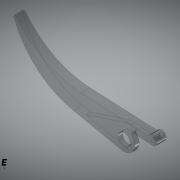
# Autodesk Inventor part: 後ろウイング先端
Saved by Autodesk Inventor 2020 (Build 240168000, 168)
## iProperties
Created: 2019-12-28
Part Number: 後ろウイング先端
Material: ポリカーボネート、クリア
Document SubType Name: Modeling
Designer: tanjihayato
Density: 1.2 g/cm^3
Appearance: ポリカーボネート - クリア
Author: tanjihayato
Autodesk Inventor part; units mm, degrees
ref_plane "YZ Plane" through (0, 0, 0) normal (1, 0, 0) x (0, 1, 0)
ref_plane "XZ Plane" through (0, 0, 0) normal (0, 1, 0) x (-1, 0, 0)
ref_plane "XY Plane" through (0, 0, 0) normal (0, 0, 1) x (1, 0, 0)
sketch "スケッチ1" plane through (0, 0, 0) normal (0, 0, 1) x (1, 0, 0)
  circle A0 centre (-145.5257, 0.5882) radius 1.5
  circle A1 centre (-139.5445, -10.0968) radius 1.5
  circle A2 centre (-105.5257, -16.4118) radius 30.1 construction
  line L0 (-170.915, -81.4118) -> (490.0044, -81.4118)
  circle A3 centre (-145.5257, 0.5882) radius 4.025
  circle A4 centre (-139.5445, -10.0968) radius 3
  circle A5 centre (-145.5257, 0.5882) radius 7.025
  line L1 (-146.2365, -6.4007) -> (-139.241, -7.1122)
  line L2 (-139.2044, 3.6529) -> (-134.6999, -5.6381)
  line L3 (-134.6999, -5.6381) -> (-136.7303, -11.1361)
  circle A6 centre (-105.5257, -16.4118) radius 31.1 construction
  line L4 (-145.1707, 7.6042) -> (-218.0775, 11.2924)
  line L5 (-145.8806, -6.4278) -> (-218.7874, -2.7396)
  circle A7 centre (-218.4324, 4.2764) radius 1.5
  circle A8 centre (-218.4324, 4.2764) radius 4.025
  circle A9 centre (-218.4324, 4.2764) radius 7.025
  circle A10 centre (-218.4324, 4.2764) radius 7.525
  line L6 (-214.5805, 10.7408) -> (-189.4684, -4.2228)
  circle A11 centre (-199.4194, 13.3524) radius 1.25
  arc A12 (-199.5709, 10.3562) -> (-202.1936, 14.494) centre (-199.4194, 13.3524) ccw
  line L7 (-202.1936, 14.494) -> (-247.2482, 16.7732)
  arc A13 (-289.8377, 39.1951) -> (-247.2482, 16.7732) centre (-244.3571, 73.9244) ccw
  arc A14 (-289.8377, 39.1951) -> (-291.571, 38.2429) centre (-290.6325, 38.5882) ccw
  arc A15 (-291.571, 38.2429) -> (-252.1456, 4.177) centre (-241.0929, 56.8157) ccw
  line L8 (-252.1456, 4.177) -> (-219.876, -2.5987)
  line L9 (-217.2943, 11.7148) -> (-212.7833, 11.0246)
  arc A16 (-212.7833, 11.0246) -> (-213.5315, 9.3094) centre (-212.8339, 10.0259) ccw
  line L10 (-220.7856, 11.424) -> (-246.4378, 2.9786)
  point P0 (0, 0)
  point P1 (0, 0)
  point P2 (0, 0)
  dimension "d17" = 6
  dimension "d18" = 8.05
  dimension "d19" = 3
  dimension "d20" = 1
  dimension "d21" = 3
  dimension "d22" = 8.05
  dimension "d23" = 3
  dimension "d24" = 0.5
  dimension "d25" = 2.5
  dimension "d26" = 6
  dimension "d27" = 2
  dimension "d28" = 120
  dimension "d29" = 4
  dimension "d30" = 150
  dimension "d31" = 1
  dimension "d32" = 73
  dimension "d33" = 79.9384
  constraints: 23 point on circle, 22 end point, 19 tangent, 16 centre point, 4 coincident, 4 point on line, 1 parallel, 4 other
  measures "d17" diameter of A4
  measures "d18" diameter of A3
  measures "d19" radial gap between concentric circles of A3 A5
  measures "d21" diameter of A7
  measures "d22" diameter of A8
  measures "d23" radial gap between concentric circles of A8 A9
  measures "d24" radial gap between concentric circles of A9 A10
  measures "d25" diameter of A11
  measures "d26" diameter of A12
  measures "d27" diameter of A14
  measures "d28" distance from line of L0 A14.centre
  measures "d29" distance between parallel lines of L4 L7
  measures "d30" distance of A14.centre A0.centre
  measures "d31" radius of A16
  measures "d32" distance of A0.centre A7.centre
  measures "d33" distance of A14.centre A7.centre
extrude "押し出し1" add sketch "スケッチ1" along normal blind 6 contours A16 A10 L6 | L6 A10 L4 A16 | L4 L9 A10 L10 L8 A15 A14 A13 L7 A12 | A9 | L8 L10 A10 | A10 L4 A9 L8 | A10 A16 A9 L4 | L4 A10 L9
extrude "押し出し2" cut sketch "スケッチ1" along normal blind 3 contours A16 A10 L6 | L6 A10 L4 A16 | A9 | L8 L10 A10 | A10 L4 A9 L8 | A10 A16 A9 L4 | L4 A10 L9
sketch "スケッチ2" plane through (0, 0, 0) normal (0, 0, -1) x (-1, 0, 0)
  circle A0 centre (199.4194, 13.3524) radius 1.25 projected
  line L0 (212.7833, 11.0246) -> (217.2943, 11.7148) projected
  arc A1 (220.7856, 11.424) -> (217.2943, 11.7148) centre (218.4324, 4.2764) ccw projected
  line L1 (220.7856, 11.424) -> (246.4378, 2.9786) projected
  line L2 (252.1456, 4.177) -> (246.4378, 2.9786) projected
  arc A2 (252.1456, 4.177) -> (291.571, 38.2429) centre (241.0929, 56.8157) ccw projected
  arc A3 (291.571, 38.2429) -> (289.8377, 39.1951) centre (290.6325, 38.5882) ccw projected
  arc A4 (247.2482, 16.7732) -> (289.8377, 39.1951) centre (244.3571, 73.9244) ccw projected
  line L3 (202.1936, 14.494) -> (247.2482, 16.7732) projected
  arc A5 (202.1936, 14.494) -> (199.5709, 10.3562) centre (199.4194, 13.3524) ccw projected
  line L4 (212.7833, 11.0246) -> (199.5709, 10.3562) projected
  line L5 (246.4378, 2.9786) -> (219.876, -2.5987) projected
  line L6 (220.7856, 11.424) -> (246.4378, 2.9786) projected
  arc A6 (220.7856, 11.424) -> (217.2943, 11.7148) centre (218.4324, 4.2764) ccw projected
  line L7 (212.7833, 11.0246) -> (217.2943, 11.7148) projected
  arc A7 (213.5315, 9.3094) -> (212.7833, 11.0246) centre (212.8339, 10.0259) ccw projected
  arc A8 (213.5315, 9.3094) -> (219.876, -2.5987) centre (218.4324, 4.2764) ccw projected
  circle A9 centre (218.4324, 4.2764) radius 4.025 projected
  arc A10 (213.5315, 9.3094) -> (212.7833, 11.0246) centre (212.8339, 10.0259) ccw projected
  arc A11 (212.7833, 11.0246) -> (220.2409, -4.3364) centre (218.4324, 4.2764) ccw
  arc A12 (246.3358, 1.1428) -> (246.4378, 2.9786) centre (246.1402, 2.0744) ccw
  line L8 (220.7856, 11.424) -> (246.4378, 2.9786) projected
  line L9 (220.2409, -4.3364) -> (246.3358, 1.1428)
  point P0 (0, 0)
  constraints: 4 point on circle, 3 tangent, 2 centre point, 2 end point, 1 coincident, 1 parallel
